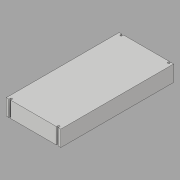
# Autodesk Inventor part: UHP-1500-230
Saved by Autodesk Inventor 2017 (Build 210142000, 142)
## iProperties
Created: 2022-09-19
Part Number: UHP-1500-230
Material: Generic
Document SubType Name: Modeling
Designer: JTS
Density: 1 g/cm^3
Appearance: Default
Author: JTS
Autodesk Inventor part; units mm, degrees
ref_plane "YZ Plane" through (0, 0, 0) normal (1, 0, 0) x (0, 1, 0)
ref_plane "XZ Plane" through (0, 0, 0) normal (0, 1, 0) x (-1, 0, 0)
ref_plane "XY Plane" through (0, 0, 0) normal (0, 0, 1) x (1, 0, 0)
sketch "Sketch1" plane through (0, 0, 0) normal (0, 0, 1) x (1, 0, 0)
  line L0 (-70, -20.5) -> (70, -20.5)
  line L1 (70, -20.5) -> (70, 20.5)
  line L2 (70, 20.5) -> (-70, 20.5)
  line L3 (-70, 20.5) -> (-70, -20.5)
  line L4 (-70, -20.5) -> (70, 20.5) construction
  line L5 (70, -20.5) -> (-70, 20.5) construction
  point P0 (0, 0)
  dimension "d0" = 140
  dimension "d1" = 41
  constraints: 12 end point, 2 horizontal, 2 midpoint, 2 vertical
  measures "d0" distance of L0.start L0.end
  measures "d1" distance of L2.end L0.start
extrude "Extrusion1" add sketch "Sketch1" along normal blind 290
sketch "Sketch2" plane through (-70, 20.5, 0) normal (0, 1, 0) x (1, 0, 0)
  line L0 (140, -290) -> (0, -290) projected
  line L1 (140, 0) -> (0, 0) projected
  arc A0 (11.25, -286) -> (6.75, -286) centre (9, -286) ccw
  arc A1 (133.25, -286) -> (128.75, -286) centre (131, -286) ccw
  arc A2 (128.75, -4) -> (133.25, -4) centre (131, -4) ccw
  arc A3 (6.75, -4) -> (11.25, -4) centre (9, -4) ccw
  line L2 (9, -286) -> (9, -4) construction
  line L3 (9, -4) -> (131, -4) construction
  line L4 (131, -4) -> (131, -286) construction
  line L5 (9, -286) -> (9, -290) construction
  line L6 (9, -4) -> (9, 0) construction
  line L7 (9, -4) -> (0, 0) construction
  line L8 (131, -4) -> (140, 0) construction
  line L9 (128.75, -286) -> (128.75, -290)
  line L10 (133.25, -286) -> (133.25, -290)
  line L11 (6.75, -286) -> (6.75, -290)
  line L12 (11.25, -286) -> (11.25, -290)
  line L13 (11.25, -4) -> (11.25, 0)
  line L14 (6.75, -4) -> (6.75, 0)
  line L15 (133.25, -4) -> (133.25, 0)
  line L16 (128.75, -4) -> (128.75, 0)
  point P0 (70, 0)
  dimension "d4" = 2.25
  dimension "d5" = 282
  dimension "d6" = 122
  constraints: 30 end point, 12 vertical, 10 point on line, 8 point on circle, 8 tangent, 4 centre point, 3 equal length, 3 equal radius, 1 coincident, 1 horizontal
  measures "d4" radius of A3
  measures "d5" distance of L2.start L2.end
  measures "d6" distance of L2.end L3.end
extrude "Extrusion2" cut sketch "Sketch2" against normal up to surface (41 mm away)
body "Solid1"
